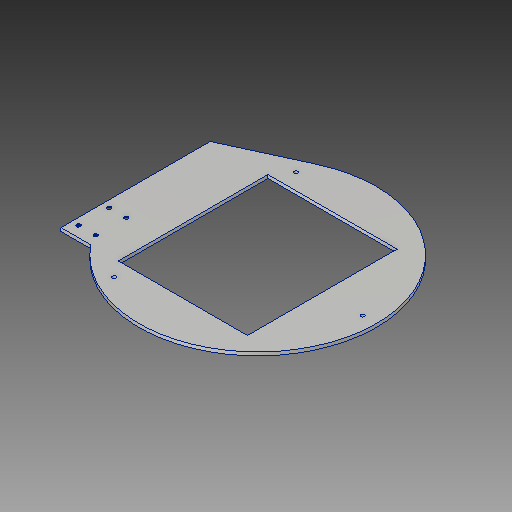
# Autodesk Inventor part: Bearing Plate
Saved by Autodesk Inventor 2019.4 (Build 234330000, 330)
## iProperties
Created: 2020-01-22
Part Number: Bearing Plate
Material: Aluminum 6061
Document SubType Name: Modeling
Designer: admin
Density: 2.7 g/cm^3
Appearance: Aluminum - Flat
Mass: 789.639 g
Surface Area: 1277.98 cm^2
Volume: 292.459 cm^3
Author: admin
Autodesk Inventor part; units mm, degrees
ref_plane "YZ Plane" through (0, 0, 0) normal (1, 0, 0) x (0, 1, 0)
ref_plane "XZ Plane" through (0, 0, 0) normal (0, 1, 0) x (-1, 0, 0)
ref_plane "XY Plane" through (0, 0, 0) normal (0, 0, 1) x (1, 0, 0)
sketch "Sketch1" plane through (0, 0, 0) normal (0, 1, 0) x (-1, 0, 0)
  arc A0 (72.9214, -159.0832) -> (136.1066, 110) centre (0, 0) ccw construction
  circle A1 centre (0, 0) radius 101.6 construction
  line L0 (-95.2, 110.3) -> (95.2, 110.3)
  line L1 (95.2, 110.3) -> (95.2, -110.3)
  line L2 (95.2, -110.3) -> (-95.2, -110.3)
  line L3 (-95.2, -110.3) -> (-95.2, 110.3)
  line L4 (-95.2, 110.3) -> (95.2, -110.3) construction
  line L5 (95.2, 110.3) -> (-95.2, -110.3) construction
  line L6 (180, 110) -> (180, -110)
  line L7 (180, -110) -> (72.9214, -159.0832)
  line L8 (180, 0) -> (0, 0)
  line L9 (180, 110) -> (136.1066, 110)
  arc A2 (136.1066, 110) -> (72.9214, -159.0832) centre (0, 0) ccw
  dimension "d0" = 350
  dimension "d1" = 203.2
  dimension "d4" = 220.6
  dimension "d5" = 190.4
  dimension "d6" = 180
  dimension "d7" = 110
  constraints: 20 end point, 4 point on circle, 3 centre point, 3 midpoint, 2 coincident, 2 horizontal, 2 parallel, 2 perpendicular, 1 tangent, 1 vertical
  measures "d0" diameter of A0
  measures "d1" diameter of A1
  measures "d4" distance of L2.end L0.start
  measures "d5" distance of L0.start L0.end
  measures "d6" distance from line of point (0, 0) L6
  measures "d7" distance from line of point (0, 0) L9
extrude "Extrusion1" add sketch "Sketch1" along normal blind 5
sketch "Sketch2" plane through (0, 0, 0) normal (0, -1, 0) x (1, 0, 0)
  circle A0 centre (-169.837, 94.1064) radius 2.0193 construction
  circle A1 centre (-169.837, 49.275) radius 2.0193 construction
  circle A2 centre (-144.437, 94.1064) radius 2.0193 construction
  circle A3 centre (-144.437, 49.275) radius 2.0193 construction
  circle A4 centre (-169.837, 94.1064) radius 3
  circle A5 centre (-144.437, 94.1064) radius 3
  circle A6 centre (-144.437, 49.275) radius 3
  circle A7 centre (-169.837, 49.275) radius 3
  point P0 (0, 0)
  dimension "d8" = 6
  dimension "d9" = 6
  dimension "d10" = 6
  dimension "d11" = 6
  constraints: 4 centre point, 4 coincident
  measures "d8" diameter of A4
  measures "d9" diameter of A5
  measures "d10" diameter of A6
  measures "d11" diameter of A7
extrude "Extrusion2" cut sketch "Sketch2" against normal through all
chamfer "Chamfer1" distance 4 angle 45 4 edges at (-172.837, 0, 49.275) (-147.437, 0, 49.275) (-172.837, 0, 94.1064) (-147.437, 0, 94.1064)
sketch "Sketch3" plane through (0, 5, 0) normal (0, 1, 0) x (1, 0, 0)
  line L0 (154.73, 0) -> (-77.365, -134.0001) construction
  line L1 (-77.365, -134.0001) -> (-77.365, 134.0001) construction
  line L2 (-77.365, 134.0001) -> (154.73, 0) construction
  circle A0 centre (-77.365, 134.0001) radius 2.75
  circle A1 centre (-77.365, -134.0001) radius 2.75
  circle A2 centre (154.73, 0) radius 2.75
  point P0 (0, 0)
  point P1 (0, 0)
  dimension "d17" = 268.0002
  dimension "d18" = 5.5
  dimension "d19" = 5.5
  dimension "d20" = 5.5
  dimension "d23" = 154.73
  constraints: 6 end point, 4 coincident, 3 centre point, 1 vertical, 7 other
  measures "d17" distance of L1.end L0.start
  measures "d18" diameter of A0
  measures "d19" diameter of A1
  measures "d20" diameter of A2
  measures "d23" distance of A2.centre point (0, 0)
extrude "Extrusion3" cut sketch "Sketch3" against normal through all
body "Solid1"
